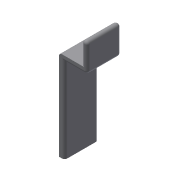
# Autodesk Inventor part: Z-Clip
Saved by Autodesk Inventor 2015 SP1 (Build 190203100, 203)
## iProperties
Created: 2015-01-15
Part Number: Z-Clip
Material: Generic
Document SubType Name: Modeling
Designer: bstevens
Density: 1 g/cm^3
Appearance: Default
Author: bstevens
Autodesk Inventor part; units mm, degrees
ref_plane "YZ Plane" through (0, 0, 0) normal (1, 0, 0) x (0, 1, 0)
ref_plane "XZ Plane" through (0, 0, 0) normal (0, 1, 0) x (-1, 0, 0)
ref_plane "XY Plane" through (0, 0, 0) normal (0, 0, 1) x (1, 0, 0)
sketch "Sketch1" plane through (0, 0, 0) normal (0, 0, 1) x (1, 0, 0)
  line L0 (0, 0) -> (0, 50.8)
  line L1 (0, 50.8) -> (12.7, 50.8)
  line L2 (12.7, 50.8) -> (12.7, 63.5)
  line L3 (12.7, 63.5) -> (15.875, 63.5)
  line L4 (15.875, 63.5) -> (15.875, 47.625)
  line L5 (15.875, 47.625) -> (3.175, 47.625)
  line L6 (3.175, 47.625) -> (3.175, 0)
  line L7 (3.175, 0) -> (0, 0)
  constraints: 16 end point, 7 perpendicular, 1 vertical
extrude "Extrusion1" add sketch "Sketch1" along normal blind 19.05
fillet "Fillet1" radius 1.5875 1 edges at (15.875, 55.5625, 19.05)
fillet "Fillet2" radius 1.5875 1 edges at (15.875, 55.5625, 0)
fillet "Fillet3" radius 1.5875 5 edges at (15.875, 63.5, 9.525) (15.41, 63.5, 18.585) (13.4938, 63.5, 19.05) (15.41, 63.5, 0.465) (13.4938, 63.5, 0)
fillet "Fillet4" radius 1.5875 5 edges at (12.7, 63.5, 9.525) (12.7, 63.035, 18.585) (12.7, 56.3563, 19.05) (12.7, 63.035, 0.465) (12.7, 56.3563, 0)
fillet "Fillet5" radius 1.5875 1 edges at (0, 50.8, 9.525)
fillet "Fillet6" radius 1.5875 1 edges at (3.175, 23.8125, 19.05)
fillet "Fillet7" radius 1.5875 5 edges at (8.7312, 47.625, 19.05) (15.41, 47.625, 18.585) (15.875, 47.625, 9.525) (15.41, 47.625, 0.465) (8.7312, 47.625, 0)
fillet "Fillet8" radius 1.5875 1 edges at (3.175, 23.8125, 0)
body "Solid1"
